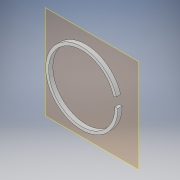
# Autodesk Inventor part: 11_Lens_Thorlabs_Mount_Ring_B
Saved by Autodesk Inventor 2019 (Build 230136000, 136)
## iProperties
Created: 2018-10-08
Part Number: 11_Lens_Thorlabs_Mount_Ring_B
Material: Generic
Document SubType Name: Modeling
Designer: diederichbenedict
Density: 1 g/cm^3
Appearance: Default
Author: diederichbenedict
Autodesk Inventor part; units mm, degrees
ref_plane "YZ Plane" through (0, 0, 0) normal (1, 0, 0) x (0, 1, 0)
ref_plane "XZ Plane" through (0, 0, 0) normal (0, 1, 0) x (-1, 0, 0)
ref_plane "XY Plane" through (0, 0, 0) normal (0, 0, 1) x (1, 0, 0)
ref_plane "Work Plane1" through (0, 0, 0) normal (0, 0, 1) x (1, 0, 0)
sketch "Sketch1" plane through (0, 0, 0) normal (0, 0, 1) x (1, 0, 0)
  circle A0 centre (-2.8988, -0.3038) radius 16.3 construction
  circle A1 centre (-2.8988, -0.3038) radius 15.6
  circle A2 centre (-2.8988, -0.3038) radius 17
  line L0 (12.6983, 0) -> (14.0985, 0)
  line L1 (12.1151, 3.932) -> (13.4417, 4.3855)
  point P0 (0, 0)
  dimension "d0" = 0.7
  dimension "d1" = 0.7
  dimension "d4" = 34
  constraints: 4 end point, 4 point on circle, 3 centre point, 1 horizontal
  measures "d0" radial gap between concentric circles of A0 A2
  measures "d1" radial gap between concentric circles of A1 A0
  measures "d4" diameter of A2
extrude "Extrusion1" add sketch "Sketch1" along normal blind 2 contours A1 L0 A2 L1 picked at (13.4719, -1.6516)
body "Solid1"
